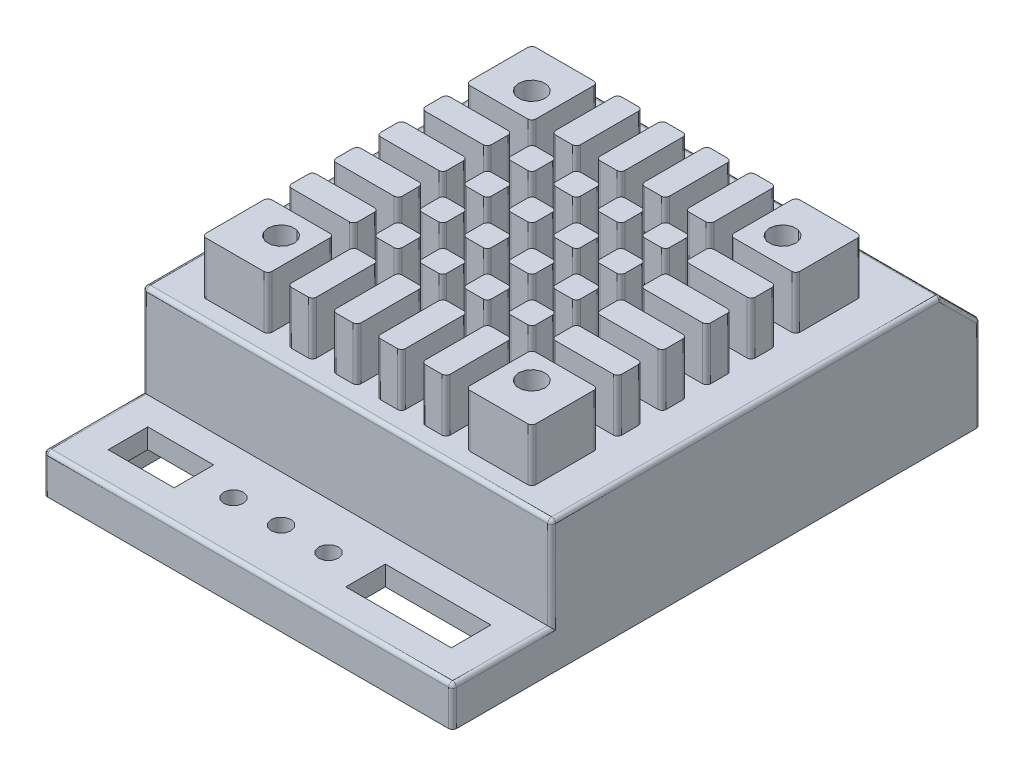
# Autodesk Inventor part: esc
Saved by Autodesk Inventor 2021 (Build 250183000, 183)
## iProperties
Created: 2021-01-20
Part Number: esc
Material: Aluminum
Document SubType Name: Modeling
Designer: User
Density: 2.7 g/cm^3
Appearance: Aluminum - Polished
Author: User
Autodesk Inventor part; units mm, degrees
ref_plane "YZ Plane" through (0, 0, 0) normal (1, 0, 0) x (0, 1, 0)
ref_plane "XZ Plane" through (0, 0, 0) normal (0, 1, 0) x (-1, 0, 0)
ref_plane "XY Plane" through (0, 0, 0) normal (0, 0, 1) x (1, 0, 0)
sketch "Sketch10" plane through (0, 0, 0) normal (1, 0, 0) x (0, 1, 0)
  line L0 (0, 0) -> (0, -40)
  line L1 (0, -40) -> (10, -40)
  line L2 (10, -40) -> (10, -7.5)
  line L3 (10, -7.5) -> (3, -7.5)
  line L4 (3, -7.5) -> (3, 0)
  line L5 (3, 0) -> (0, 0)
  dimension "d69" = 40
  dimension "d70" = 7.5
  dimension "d71" = 3
  dimension "d72" = 10
  constraints: 12 end point, 5 perpendicular, 1 coincident, 1 vertical alignment
  measures "d69" distance of L0.start L0.end
  measures "d70" distance between parallel lines of L5 L3
  measures "d71" distance between parallel lines of L0 L4
  measures "d72" distance between parallel lines of L0 L2
extrude "Extrusion10" add sketch "Sketch10" along normal mid plane 31
sketch "Sketch11" plane through (-15.5, 10, -7.5) normal (0, 1, 0) x (1, 0, 0)
  line L0 (3, 1.5) -> (28, 1.5)
  line L1 (28, 1.5) -> (28, 26.5)
  line L2 (28, 26.5) -> (3, 26.5)
  line L3 (3, 26.5) -> (3, 1.5)
  line L4 (0, 0) -> (31, 0) projected
  line L5 (31, 32.5) -> (31, 0) projected
  line L6 (0, 32.5) -> (31, 32.5) projected
  line L7 (0, 0) -> (0, 32.5) projected
  point P0 (15.5, -7.5)
  dimension "d75" = 25
  dimension "d76" = 25
  dimension "d77" = 31
  dimension "d78" = 32.5
  dimension "d79" = 3
  dimension "d80" = 1.5
  constraints: 8 end point, 2 parallel, 1 horizontal, 1 perpendicular
  measures "d75" distance of L2.end L1.end
  measures "d76" distance of L1.end L0.end
  measures "d77" distance of L6.start L5.start
  measures "d78" distance of L4.start L6.start
  measures "d79" distance between parallel lines of L7 L3
  measures "d80" distance between parallel lines of L4 L0
extrude "Extrusion11" add sketch "Sketch11" along normal blind 4 contours L3 L2 L1 L0
chamfer "Chamfer2" distance 3 angle 45 1 edges at (0, 10, -40)
sketch "Sketch12" plane through (12.5, 10, -9) normal (1, 0, 0) x (0, 0, -1)
  line L0 (0, 0) -> (25, 0) projected
  line L1 (5, 4) -> (6.5, 4)
  line L2 (6.5, 4) -> (6.5, 0)
  line L3 (6.5, 0) -> (5, 0)
  line L4 (5, 0) -> (5, 4)
  line L5 (0, 4) -> (25, 4) projected
  line L6 (8.375, 0) -> (8.375, 4)
  line L7 (8.375, 4) -> (9.875, 4)
  line L8 (9.875, 4) -> (9.875, 0)
  line L9 (9.875, 0) -> (8.375, 0)
  line L10 (11.75, 0) -> (11.75, 4)
  line L11 (11.75, 4) -> (13.25, 4)
  line L12 (13.25, 4) -> (13.25, 0)
  line L13 (13.25, 0) -> (11.75, 0)
  line L14 (15.125, 0) -> (15.125, 4)
  line L15 (15.125, 4) -> (16.625, 4)
  line L16 (16.625, 4) -> (16.625, 0)
  line L17 (16.625, 0) -> (15.125, 0)
  line L18 (18.5, 0) -> (18.5, 4)
  line L19 (18.5, 4) -> (20, 4)
  line L20 (20, 4) -> (20, 0)
  line L21 (20, 0) -> (18.5, 0)
  line L22 (0, 0) -> (0, 4) projected
  line L23 (25, 0) -> (25, 4) projected
  point P0 (-9, -10)
  point P1 (20, 0)
  point P2 (18.5, 4)
  point P3 (18.5, 0)
  point P4 (16.625, 0)
  point P5 (15.125, 4)
  point P6 (15.125, 0)
  point P7 (13.25, 0)
  point P8 (11.75, 4)
  point P9 (11.75, 0)
  point P10 (9.875, 0)
  point P11 (9.875, 4)
  point P12 (8.375, 4)
  point P13 (8.375, 0)
  point P14 (6.5, 4)
  point P15 (5, 4)
  point P16 (5, 0)
  dimension "d88" = 3.375
  dimension "d93" = 5
  dimension "d94" = 1.5
  dimension "d95" = 5
  constraints: 40 end point, 2 horizontal, 2 parallel, 1 horizontal alignment, 1 perpendicular, 1 point on line, 32 other
  measures "d88" distance of L3.end L6.start
  measures "d93" distance between parallel lines of L22 L4
  measures "d94" distance between parallel lines of L4 L2
  measures "d95" distance between parallel lines of L23 L20
extrude "Extrusion12" cut sketch "Sketch12" against normal up to surface (25 mm away) contours L4 L1 L2 L0 | L6 L5 L8 L0 | L10 L5 L12 L0 | L14 L5 L16 L0 | L18 L5 L20 L0
sketch "Sketch13" plane through (-12.5, 10, -9) normal (0, 0, 1) x (1, 0, 0)
  line L0 (0, 4) -> (25, 4) projected
  line L1 (25, 0) -> (0, 0) projected
  line L2 (5, 4) -> (6.5, 4)
  line L3 (6.5, 4) -> (6.5, 0)
  line L4 (6.5, 0) -> (5, 0)
  line L5 (5, 0) -> (5, 4)
  line L6 (8.375, 0) -> (8.375, 4)
  line L7 (8.375, 4) -> (9.875, 4)
  line L8 (9.875, 4) -> (9.875, 0)
  line L9 (9.875, 0) -> (8.375, 0)
  line L10 (11.75, 0) -> (11.75, 4)
  line L11 (11.75, 4) -> (13.25, 4)
  line L12 (13.25, 4) -> (13.25, 0)
  line L13 (13.25, 0) -> (11.75, 0)
  line L14 (15.125, 0) -> (15.125, 4)
  line L15 (15.125, 4) -> (16.625, 4)
  line L16 (16.625, 4) -> (16.625, 0)
  line L17 (16.625, 0) -> (15.125, 0)
  line L18 (18.5, 0) -> (18.5, 4)
  line L19 (18.5, 4) -> (20, 4)
  line L20 (20, 4) -> (20, 0)
  line L21 (20, 0) -> (18.5, 0)
  line L22 (0, 0) -> (0, 4) projected
  line L23 (25, 0) -> (25, 4) projected
  point P0 (12.5, -10)
  point P1 (20, 0)
  point P2 (18.5, 0)
  point P3 (16.625, 0)
  point P4 (15.125, 0)
  point P5 (13.25, 0)
  point P6 (11.75, 0)
  point P7 (9.875, 0)
  point P8 (8.375, 0)
  point P9 (5, 0)
  dimension "d100" = 3.375
  dimension "d105" = 5
  dimension "d106" = 1.5
  dimension "d107" = 5
  constraints: 40 end point, 2 horizontal, 2 parallel, 2 point on line, 1 perpendicular, 32 other
  measures "d100" distance of L4.end L6.start
  measures "d105" distance between parallel lines of L22 L5
  measures "d106" distance between parallel lines of L5 L3
  measures "d107" distance between parallel lines of L23 L20
extrude "Extrusion13" cut sketch "Sketch13" against normal up to surface (25 mm away) contours L0 L3 L1 L5 | L0 L8 L1 L6 | L0 L12 L1 L10 | L0 L16 L1 L14 | L0 L20 L1 L18
sketch "Sketch15" plane through (-15.5, 3, 0) normal (0, 1, 0) x (1, 0, 0)
  line L0 (28.5, 2.4) -> (20.5, 2.4)
  line L1 (20.5, 2.4) -> (20.5, 5.4)
  line L2 (20.5, 5.4) -> (28.5, 5.4)
  line L3 (28.5, 5.4) -> (28.5, 2.4)
  line L4 (7.5, 2.4) -> (2.5, 2.4)
  line L5 (2.5, 2.4) -> (2.5, 5.4)
  line L6 (2.5, 5.4) -> (7.5, 5.4)
  line L7 (7.5, 5.4) -> (7.5, 2.4)
  circle A0 centre (10.4, 4) radius 0.75
  line L8 (0, 0) -> (31, 0) projected
  line L9 (31, 7.5) -> (31, 0) projected
  line L10 (0, 7.5) -> (31, 7.5) projected
  line L11 (0, 0) -> (0, 7.5) projected
  circle A1 centre (14, 4) radius 0.75
  circle A2 centre (17.6, 4) radius 0.75
  point P0 (15.5, 0)
  dimension "d120" = 3.6
  dimension "d125" = 2.5
  dimension "d126" = 2.4
  dimension "d127" = 3
  dimension "d128" = 8
  dimension "d129" = 1.5
  dimension "d130" = 3
  dimension "d131" = 5
  dimension "d132" = 2.5
  dimension "d134" = 4
  dimension "d143" = 13
  dimension "d144" = 2.9
  dimension "d145" = 7.2
  constraints: 16 end point, 4 parallel, 3 centre point, 3 horizontal, 2 perpendicular, 1 point on line, 4 other
  measures "d120" distance of A0.centre A1.centre
  measures "d125" distance between parallel lines of L9 L3
  measures "d126" distance between parallel lines of L8 L0
  measures "d127" distance of L2.end L0.start
  measures "d128" distance of L0.start L0.end
  measures "d129" diameter of A0
  measures "d130" distance of L4.end L5.end
  measures "d131" distance of L4.start L4.end
  measures "d132" distance between parallel lines of L11 L5
  measures "d134" distance from line of L8 A0.centre
  measures "d143" distance between parallel lines of L1 L7
  measures "d144" distance from line of L7 A0.centre
  measures "d145" distance of A2.centre A0.centre
extrude "Extrusion14" cut sketch "Sketch15" against normal up to surface (3 mm away) contours L0 L1 L2 L3 | L4 L5 L6 L7 | A0 | A1 | A2
sketch "Sketch16" plane through (15.5, 0, -40) normal (0, 0, -1) x (-1, 0, 0)
  line L0 (0, 0) -> (31, 0) projected
  line L1 (2, 0) -> (29, 0)
  line L2 (29, 0) -> (29, 1.5)
  line L3 (29, 1.5) -> (2, 1.5)
  line L4 (2, 1.5) -> (2, 0)
  line L5 (0, 0) -> (0, 7) projected
  point P0 (15.5, 0)
  point P1 (29, 0)
  dimension "d137" = 1.5
  dimension "d138" = 27
  dimension "d139" = 31
  dimension "d140" = 2
  constraints: 8 end point, 2 parallel, 1 horizontal, 1 perpendicular, 1 point on line
  measures "d137" distance of L2.end L1.end
  measures "d138" distance of L2.end L3.end
  measures "d139" distance of L0.start L0.end
  measures "d140" distance between parallel lines of L5 L4
extrude "Extrusion15" cut sketch "Sketch16" against normal blind 38
sketch "Sketch17" plane through (-15.5, 14, -7.5) normal (0, 1, 0) x (1, 0, 0)
  line L0 (8, 1.5) -> (8, 6.5) projected
  line L1 (8, 6.5) -> (3, 6.5) projected
  line L2 (3, 6.5) -> (3, 1.5) projected
  line L3 (3, 1.5) -> (8, 1.5) projected
  line L4 (8, 21.5) -> (8, 26.5) projected
  line L5 (8, 26.5) -> (3, 26.5) projected
  line L6 (3, 26.5) -> (3, 21.5) projected
  line L7 (3, 21.5) -> (8, 21.5) projected
  line L8 (23, 26.5) -> (23, 21.5) projected
  line L9 (23, 21.5) -> (28, 21.5) projected
  line L10 (28, 21.5) -> (28, 26.5) projected
  line L11 (28, 26.5) -> (23, 26.5) projected
  line L12 (23, 6.5) -> (23, 1.5) projected
  line L13 (23, 1.5) -> (28, 1.5) projected
  line L14 (28, 1.5) -> (28, 6.5) projected
  line L15 (28, 6.5) -> (23, 6.5) projected
  circle A0 centre (6, 4.5) radius 1
  circle A1 centre (6, 23.5) radius 1
  circle A2 centre (25, 4.5) radius 1
  circle A3 centre (25, 23.5) radius 1
  point P0 (15.5, -7.5)
  dimension "d146" = 2
  dimension "d147" = 3
  dimension "d148" = 3
  dimension "d149" = 25
  dimension "d150" = 25
  dimension "d153" = 19
  dimension "d156" = 19
  constraints: 4 centre point, 1 horizontal, 1 vertical, 6 other
  measures "d146" diameter of A0
  measures "d147" distance from line of L2 A0.centre
  measures "d148" distance from line of L3 A0.centre
  measures "d149" distance between parallel lines of L5 L3
  measures "d150" distance between parallel lines of L14 L2
  measures "d153" distance of A0.centre A1.centre
  measures "d156" distance of A0.centre A2.centre
extrude "Extrusion16" cut sketch "Sketch17" against normal up to surface (12.5 mm away) contours A0 | A1 | A2 | A3
fillet "Fillet6" radius 0.3 161 edges at (-15.5, 3.5, -40) (0, 7, -40) (15.5, 3.5, -40) (-0.75, 12, -27.5) (-0.75, 12, -25.625) (-0.75, 12, -29) (-0.75, 12, -34) (-0.75, 12, -22.25) (-0.75, 12, -24.125) (-0.75, 12, -18.875) (-0.75, 12, -20.75) (-0.75, 12, -15.5) (-0.75, 12, -17.375) (-0.75, 12, -14) (-0.75, 12, -9) (0.75, 12, -27.5) (0.75, 12, -25.625) (0.75, 12, -29) (0.75, 12, -34) (0.75, 12, -22.25) (0.75, 12, -24.125) (0.75, 12, -18.875) (0.75, 12, -20.75) (0.75, 12, -15.5) (0.75, 12, -17.375) (0.75, 12, -14) (0.75, 12, -9) (-6, 12, -22.25) (-6, 12, -24.125) (-6, 12, -27.5) (-6, 12, -25.625) (-6, 12, -29) (-6, 12, -34) (-6, 12, -18.875) (-6, 12, -20.75) (-6, 12, -15.5) (-6, 12, -17.375) (-7.5, 12, -27.5) (-7.5, 12, -25.625) (-7.5, 12, -29) (-7.5, 12, -34) (-7.5, 12, -22.25) (-7.5, 12, -24.125) (-7.5, 12, -18.875) (-7.5, 12, -20.75) (-7.5, 12, -15.5) (-7.5, 12, -17.375) (-7.5, 12, -14) (-7.5, 12, -9) (-6, 12, -14) (-6, 12, -9) (7.5, 12, -22.25) (7.5, 12, -24.125) (7.5, 12, -27.5) (7.5, 12, -25.625) (7.5, 12, -29) (7.5, 12, -34) (7.5, 12, -18.875) (7.5, 12, -20.75) (7.5, 12, -15.5) (7.5, 12, -17.375) (6, 12, -27.5) (6, 12, -25.625) (6, 12, -29) (6, 12, -34) (6, 12, -22.25) (6, 12, -24.125) (6, 12, -18.875) (6, 12, -20.75) (6, 12, -15.5) (6, 12, -17.375) (6, 12, -14) (6, 12, -9) (7.5, 12, -14) (7.5, 12, -9) (-4.125, 12, -27.5) (-4.125, 12, -25.625) (-4.125, 12, -29) (-4.125, 12, -34) (-4.125, 12, -22.25) (-4.125, 12, -24.125) (-4.125, 12, -18.875) (-4.125, 12, -20.75) (-4.125, 12, -15.5) (-4.125, 12, -17.375) (-4.125, 12, -14) (-4.125, 12, -9) (-2.625, 12, -27.5) (-2.625, 12, -25.625) (-2.625, 12, -29) (-2.625, 12, -34) (-2.625, 12, -22.25) (-2.625, 12, -24.125) (-2.625, 12, -18.875) (-2.625, 12, -20.75) (-2.625, 12, -15.5) (-2.625, 12, -17.375) (-2.625, 12, -14) (-2.625, 12, -9) (4.125, 12, -22.25) (4.125, 12, -24.125) (4.125, 12, -27.5) (4.125, 12, -25.625) (4.125, 12, -29) (4.125, 12, -34) (4.125, 12, -18.875) (4.125, 12, -20.75) (4.125, 12, -15.5) (4.125, 12, -17.375) (2.625, 12, -27.5) (2.625, 12, -25.625) (2.625, 12, -29) (2.625, 12, -34) (2.625, 12, -22.25) (2.625, 12, -24.125) (2.625, 12, -18.875) (2.625, 12, -20.75) (2.625, 12, -15.5) (2.625, 12, -17.375) (2.625, 12, -14) (2.625, 12, -9) (4.125, 12, -14) (4.125, 12, -9) (-12.5, 12, -9) (12.5, 12, -9) (-12.5, 12, -14) (12.5, 12, -14) (-12.5, 12, -15.5) (12.5, 12, -15.5) (-12.5, 12, -17.375) (12.5, 12, -17.375) (-12.5, 12, -18.875) (12.5, 12, -18.875) (12.5, 12, -34) (-12.5, 12, -34) (-12.5, 12, -20.75) (12.5, 12, -20.75) (12.5, 12, -29) (-12.5, 12, -29) (-12.5, 12, -22.25) (12.5, 12, -22.25) (12.5, 12, -27.5) (-12.5, 12, -27.5) (-12.5, 12, -24.125) (12.5, 12, -24.125) (0, 10, -37) (-15.5, 10, -22.25) (0, 10, -7.5) (15.5, 10, -22.25) (12.5, 12, -25.625) (-12.5, 12, -25.625) (15.5, 8.5, -38.5) (-15.5, 8.5, -38.5) (-15.5, 1.5, 0) (-15.5, 3, -3.75) (-15.5, 6.5, -7.5) (15.5, 1.5, 0) (0, 3, 0) (15.5, 3, -3.75) (15.5, 6.5, -7.5) (13.5, 0.75, -2)
equation "\"d79\" = -0.5 * d75 + 0.5 * d77"
body "Solid3"
